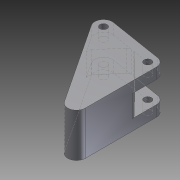
# Autodesk Inventor part: GHI
Saved by Autodesk Inventor 2011 SP2 (Build 150309200, 309)
## iProperties
Created: 2014-05-09
Part Number: GHI
Document SubType Name: Modeling
Designer: Maurice Woods
Density: 1 g/cm^3
ScaleFactor: 1.000 ul
LengthA: 1.000 in
LengthB: 1.092 in
LengthC: 1.034 in
LengthD: 1.055 in
LengthE: 1.468 in
LengthF: 1.037 in
LengthG: 0.966 in
LengthH: 1.729 in
LengthI: 1.289 in
LengthJ: 1.316 in
LengthK: 1.500 in
LengthL: 0.205 in
LengthM: 0.395 in
d0_1: 1.000 in
d1: 1.316 in
d2: 0.395 in
d3: 0.205 in
d4: 1.092 in
d5: 1.034 in
d7: 1.055 in
d8: 1.468 in
d9: 1.037 in
d10: 0.966 in
d11: 1.729 in
d12: 1.289 in
d13: 1.500 in
Author: Maurice Woods
Autodesk Inventor part; units mm, degrees
ref_plane "YZ Plane" through (0, 0, 0) normal (1, 0, 0) x (0, 1, 0)
ref_plane "XZ Plane" through (0, 0, 0) normal (0, 1, 0) x (-1, 0, 0)
ref_plane "XY Plane" through (0, 0, 0) normal (0, 0, 1) x (1, 0, 0)
sketch "Sketch1" plane through (0, 0, 0) normal (0, 0, 1) x (1, 0, 0)
  line L0 (0, 0) -> (-24.2225, 3.8783) construction
  line L1 (-24.2225, 3.8783) -> (0, -32.7525) construction
  line L2 (0, -32.7525) -> (0, 0) construction
  line L3 (0.6324, 3.9497) -> (-23.5901, 7.828)
  line L4 (-27.559, 1.672) -> (-3.3365, -34.9588)
  line L5 (4, -32.7525) -> (4, 0)
  arc A0 (-23.5901, 7.828) -> (-27.559, 1.672) centre (-24.2225, 3.8783) ccw
  arc A1 (4, 0) -> (0.6324, 3.9497) centre (0, 0) ccw
  arc A2 (-3.3365, -34.9588) -> (4, -32.7525) centre (0, -32.7525) ccw
  dimension "d0" = 32.7525
  dimension "d6" = 24.531
  dimension "d14" = 43.9153
  dimension "d15" = 4
  constraints: 12 end point, 6 point on circle, 6 tangent, 3 centre point, 2 coincident, 2 equal radius, 1 vertical, 2 other
  measures "d0" distance of L1.end L0.start
  measures "d6" distance of L0.start L0.end
  measures "d14" distance of L0.end L1.end
  measures "d15" radius of A0
extrude "Extrusion1" add sketch "Sketch1" along normal mid plane 20
sketch "Sketch2" plane through (0, 0, 0) normal (0, 0, 1) x (1, 0, 0)
  arc A0 (-23.5901, 7.828) -> (-27.559, 1.672) centre (-24.2225, 3.8783) ccw construction
  line L0 (-3.3365, -34.9588) -> (-27.559, 1.672) construction
  arc A1 (-3.3365, -34.9588) -> (4, -32.7525) centre (0, -32.7525) ccw construction
  line L1 (4, 0) -> (4, -32.7525) construction
  arc A2 (4, 0) -> (0.6324, 3.9497) centre (0, 0) ccw construction
  line L2 (-23.5901, 7.828) -> (0.6324, 3.9497) construction
  arc A3 (4, 0) -> (0.6324, 3.9497) centre (0, 0) ccw
  line L3 (4, 0) -> (4, -10.3073)
  arc A4 (-3.3365, -34.9588) -> (4, -32.7525) centre (0, -32.7525) ccw construction
  line L4 (-3.3365, -34.9588) -> (-7.3441, -28.8984) construction
  arc A5 (-23.5901, 7.828) -> (-27.559, 1.672) centre (-24.2225, 3.8783) ccw
  line L5 (-23.5901, 7.828) -> (-14.2736, 6.3363)
  line L6 (-24.408, -3.0932) -> (-14.2736, 6.3363)
  line L7 (-11.9287, 5.9609) -> (4, -10.3073)
  line L8 (-7.3441, -28.8984) -> (4, -26.0222) construction
  line L9 (-24.408, -3.0932) -> (-27.559, 1.672)
  line L10 (-7.3441, -28.8984) -> (-24.408, -3.0932) construction
  line L11 (4, -10.3073) -> (4, -26.0222) construction
  line L12 (4, -26.0222) -> (4, -32.7525) construction
  line L13 (-11.9287, 5.9609) -> (0.6324, 3.9497)
  line L14 (-14.2736, 6.3363) -> (-11.9287, 5.9609) construction
  constraints: 24 end point, 8 collinear, 6 point on circle, 3 centre point, 3 concentric, 1 point on line
extrude "Extrusion2" cut sketch "Sketch2" along normal mid plane 10
fillet "Fillet1" radius 2 4 edges at (4, -10.3073, 0) (-11.9287, 5.9609, 0) (-24.408, -3.0932, 0) (-14.2736, 6.3363, 0)
sketch "Sketch3" plane through (0, 0, 10) normal (0, 0, 1) x (1, 0, 0)
  arc A0 (-23.5901, 7.828) -> (-27.559, 1.672) centre (-24.2225, 3.8783) ccw construction
  arc A1 (-3.3365, -34.9588) -> (4, -32.7525) centre (0, -32.7525) ccw construction
  arc A2 (4, 0) -> (0.6324, 3.9497) centre (0, 0) ccw construction
hole "Hole1" at (-24.2225, 3.8783, 10) at (0, 0, 10) direction (0, 0, -1) diameter 3.4 end through all clearance for "Socket Head Cap Screw" size "M3" standard "Ansi Metric M Profile"
equation "\"d0\" = LengthI"
equation "\"d6\" = LengthG"
equation "\"d14\" = LengthH"
equation "\"LengthI\" = 32.752538"
equation "\"LengthG\" = 24.531041"
equation "\"LengthH\" = 43.915254"
body "Solid1"
